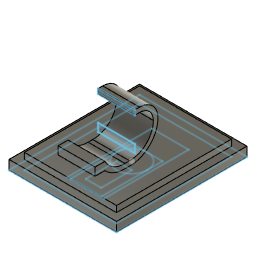
Keyhook (Autodesk Fusion 360 design; units mm, degrees)
Autodesk Fusion 360 part; units mm, degrees
note: some values were not read from the file. Set by a fixed rule: which sketch regions a step uses.
sketch "Sketch1" plane through (0, 0, 0) normal (0, 0, 1) x (1, 0, 0)
  line L0 (-35, 50) -> (35, 50)
  line L1 (35, 50) -> (35, -35)
  line L2 (35, -35) -> (-35, -35)
  line L3 (-35, -35) -> (-35, 50)
  line L4 (-10, -20) -> (10, -20)
  line L5 (10, -20) -> (10, 20)
  line L6 (10, 20) -> (-10, 20)
  line L7 (-10, 20) -> (-10, -20)
  circle A0 centre (0, 10) radius 10
  line L8 (-5, -15) -> (5, -15)
  line L9 (5, -15) -> (5, 5)
  line L10 (5, 5) -> (-5, 5)
  line L11 (-5, 5) -> (-5, -15)
  line L12 (-30, -30) -> (30, -30)
  line L13 (30, -30) -> (30, 45)
  line L14 (30, 45) -> (-30, 45)
  line L15 (-30, 45) -> (-30, -30)
  line L16 (-12, 35) -> (12, 35)
  line L17 (12, 35) -> (12, -20)
  line L18 (12, -20) -> (-12, -20)
  line L19 (-12, -20) -> (-12, 35)
  constraint horizontal L0
  constraint vertical L1
  constraint horizontal L2
  constraint vertical L3
  constraint horizontal L4
  constraint vertical L5
  constraint horizontal L6
  constraint vertical L7
  constraint tangent L6 A0
  constraint horizontal L8
  constraint vertical L9
  constraint horizontal L10
  constraint vertical L11
  constraint horizontal L12
  constraint vertical L13
  constraint horizontal L14
  constraint vertical L15
  constraint horizontal L16
  constraint vertical L17
  constraint horizontal L18
  constraint vertical L19
extrude "Extrude1" add sketch "Sketch1" along normal blind 10 contours L0 L1 L2 L3 | L4 L5 L7 A0 L8 L9 L11 L18 | L5 L6 L7 L16 L17 L18 L19 | L6 L7 A0 | A0 L9 L10 L11 | L5 L6 A0 | A0 L9 L10 L11 | A0 L8 L9 L11 | L12 L13 L14 L15 makes body 1
extrude "Extrude2" cut sketch "Sketch1" along normal blind 8 contours L4 L5 L7 A0 L8 L9 L11 L18 | L6 L7 A0 | A0 L9 L10 L11 | L5 L6 A0 | A0 L9 L10 L11 | A0 L8 L9 L11 bodies 1
extrude "Extrude3" add sketch "Sketch1" along normal blind 3.5 contours L4 L5 L7 A0 L8 L9 L11 L18 | L6 L7 A0 | L5 L6 A0 bodies 1
extrude "Extrude4" cut 1 faces at (-11.6667, 21.6667, 10) along direction (0, 0, -1) blind 3 on bodies 1 bodies 1
extrude "Extrude5" add sketch "Sketch1" 1 faces at (-0.2491, 39.9907, 0) along normal blind 10 and the other way blind -7 contours L0 L1 L2 L3 | L4 L5 L7 A0 L8 L9 L11 L18 | L5 L6 L7 L16 L17 L18 L19 | L6 L7 A0 | A0 L9 L10 L11 | L5 L6 A0 | A0 L9 L10 L11 | A0 L8 L9 L11 | L12 L13 L14 L15 on bodies 1 bodies 1
extrude "Extrude6" cut sketch "Sketch1" along normal blind 10 and the other way blind -6 contours L0 L1 L2 L3 bodies 1
extrude "Extrude7" add sketch "Sketch1" along normal blind 20 and the other way blind -6 contours L4 L5 L7 A0 L8 L9 L11 L18 | L5 L6 L7 L16 L17 L18 L19 | L6 L7 A0 | A0 L9 L10 L11 | L5 L6 A0 | A0 L9 L10 L11 | A0 L8 L9 L11 bodies 1
sketch "Sketch2" plane through (0, 0, 0) normal (1, 0, 0) x (0, 1, 0)
  circle A0 centre (-7, 27) radius 14
  circle A1 centre (-7, 27) radius 17
  line L0 (-19.5016, 20.6984) -> (-19.5016, 15.48)
  circle A2 centre (-3, 28) radius 15
  circle A3 centre (-3, 28) radius 18
  circle A4 centre (3, 28) radius 9
  circle A5 centre (3, 28) radius 12
  line L1 (2.8002, 36.9978) -> (2.8002, 39.9983)
  line L2 (-7.5099, 10.0076) -> (-2.4753, 10.0076)
  line L3 (-2.4753, 13.0092) -> (-7.5069, 13.0092)
  dimension "d21" = 28
  dimension "d22" = 34
  dimension "d23" = 30
  dimension "d24" = 36
  dimension "d25" = 18
  dimension "d26" = 24
  constraint concentric A0 A1
  constraint coincident A0 L0.start
  constraint coincident A1 L0.end
  constraint vertical L0
  constraint concentric A2 A3
  constraint concentric A4 A5
  constraint coincident A0 L1.start
  constraint coincident A4 L1.start
  constraint coincident A5 L1.end
  constraint vertical L1
  constraint coincident A1 L2.start
  constraint coincident A3 L2.end
  constraint horizontal L2
  constraint coincident A2 L3.start
  constraint coincident A0 L3.end
  constraint parallel L2 L3
  measures "d21" diameter of A0
  measures "d22" diameter of A1
  measures "d23" diameter of A2
  measures "d24" diameter of A3
  measures "d25" diameter of A4
  measures "d26" diameter of A5
delete_face "DeleteFace1" 1 faces at (12, 16.6667, 13.3333) on bodies 1
extrude "Extrude8" add sketch "Sketch2" along normal mid plane 24 separate body contours A1 A4 A5 L1 | A1 A2 A4 A5 | A2 A5 | A1 A2 A3 A5 L2 | A0 A1 A2 A3 L3 | A0 A1 L0 A3 L2 | A1 A3 L2 | A3 L2 picked at (8.4808, 36.5991) makes body 2
sketch "Sketch5" plane through (0, 0, 0) normal (0, 1, 0) x (1, 0, 0)
  line L0 (-12, -40) -> (12, -40)
  line L1 (12, -40) -> (12, -37)
  line L2 (12, -37) -> (-12, -37)
  line L3 (-12, -37) -> (-12, -40)
  line L4 (12, -15.5) -> (-11.9996, -15.5)
  line L5 (-11.9996, -15.5) -> (-11.9996, -20.7026)
  line L6 (-11.9996, -20.7026) -> (12, -20.7026)
  line L7 (12, -20.7026) -> (12, -15.5)
  constraint horizontal L0
  constraint vertical L1
  constraint horizontal L2
  constraint vertical L3
  constraint horizontal L4
  constraint vertical L5
  constraint horizontal L6
  constraint vertical L7
extrude "Extrude9" add sketch "Sketch5" along normal blind 3 contours L0 L1 L2 L3 bodies 2
extrude "Extrude10" add sketch "Sketch5" along normal blind -26 and the other way blind 19.5 contours L4 L5 L6 L7 bodies 2
